Autodesk Fusion 360 part; units mm, degrees
(part 8 of 8)
equation "d2179 = ( BaseY + Depth - 12 mm )"
equation "d2180 = -( -( UpperDeckHeight - PanHeight - 8 mm ) )"
equation "d2181 = TowerFrame"
equation "d2183 = UpperDeckHeight - PanHeight"
equation "d2185 = ( BaseX ) + ( ( TowerFrame - 5 mm ) / 2 )"
equation "d2186 = ( BaseY + 8 mm ) - ( 2.5 mm )"
equation "d2189 = PegHeight"
equation "d2191 = UpperDeckHeight - PanHeight"
equation "d2193 = ( BaseX ) + ( ( TowerFrame - 5 mm ) / 2 )"
equation "d2194 = ( BaseY + Depth - 8 mm ) - ( 2.5 mm )"
equation "d2197 = PegHeight"
equation "d2201 = BaseX + TowerWidth - TowerFrame"
equation "d2202 = BaseY"
equation "d2203 = TowerFrame"
equation "d2204 = Depth"
equation "d2205 = UpperDeckHeight - PanHeight"
equation "d2207 = BaseX + TowerWidth - TowerFrame"
equation "d2209 = -( -( 8 mm ) )"
equation "d2210 = ( BaseY + 12 mm )"
equation "d2211 = ( BaseY + Depth - 12 mm )"
equation "d2212 = -( -( UpperDeckHeight - PanHeight - 8 mm ) )"
equation "d2213 = TowerFrame"
equation "d2215 = UpperDeckHeight - PanHeight"
equation "d2217 = ( BaseX + TowerWidth - TowerFrame ) + ( ( TowerFrame - 5 mm ) / 2 )"
equation "d2218 = ( BaseY + 8 mm ) - ( 2.5 mm )"
equation "d2221 = PegHeight"
equation "d2223 = UpperDeckHeight - PanHeight"
equation "d2225 = ( BaseX + TowerWidth - TowerFrame ) + ( ( TowerFrame - 5 mm ) / 2 )"
equation "d2226 = ( BaseY + Depth - 8 mm ) - ( 2.5 mm )"
equation "d2229 = PegHeight"
equation "d2231 = UpperDeckHeight - PanHeight"
equation "d2233 = ( BaseX + ( TowerFrame - 5 mm ) / 2 ) - ( FitClearance )"
equation "d2234 = ( BaseY + 8 mm ) - ( 2.5 mm + FitClearance )"
equation "d2235 = 5 mm + 2 * FitClearance"
equation "d2236 = 5 mm + 2 * FitClearance"
equation "d2237 = PegHeight + 0.3 mm"
equation "d2239 = UpperDeckHeight - PanHeight"
equation "d2241 = ( BaseX + ( TowerFrame - 5 mm ) / 2 ) - ( FitClearance )"
equation "d2242 = ( BaseY + Depth - 8 mm ) - ( 2.5 mm + FitClearance )"
equation "d2243 = 5 mm + 2 * FitClearance"
equation "d2244 = 5 mm + 2 * FitClearance"
equation "d2245 = PegHeight + 0.3 mm"
equation "d2247 = UpperDeckHeight - PanHeight"
equation "d2249 = ( BaseX + TowerWidth - TowerFrame + ( TowerFrame - 5 mm ) / 2 ) - ( FitClearance )"
equation "d2250 = ( BaseY + 8 mm ) - ( 2.5 mm + FitClearance )"
equation "d2251 = 5 mm + 2 * FitClearance"
equation "d2252 = 5 mm + 2 * FitClearance"
equation "d2253 = PegHeight + 0.3 mm"
equation "d2255 = UpperDeckHeight - PanHeight"
equation "d2257 = ( BaseX + TowerWidth - TowerFrame + ( TowerFrame - 5 mm ) / 2 ) - ( FitClearance )"
equation "d2258 = ( BaseY + Depth - 8 mm ) - ( 2.5 mm + FitClearance )"
equation "d2259 = 5 mm + 2 * FitClearance"
equation "d2260 = 5 mm + 2 * FitClearance"
equation "d2261 = PegHeight + 0.3 mm"
equation "d2265 = BaseX + LeftRun + FaucetGap + RightRun + 20 mm + 0 mm"
equation "d2266 = BaseY"
equation "d2273 = ( BaseX + LeftRun + FaucetGap + RightRun + 20 mm + 0 mm ) + ( ( 24 mm - ( PegSize + 2 * ( FitClearance - 0.05 mm ) ) ) / 2 )"
equation "d2274 = BaseY + ( 24 mm - ( PegSize + 2 * ( FitClearance - 0.05 mm ) ) ) / 2"
equation "d2275 = PegSize + 2 * ( FitClearance - 0.05 mm )"
equation "d2276 = PegSize + 2 * ( FitClearance - 0.05 mm )"
equation "d2277 = PegHeight + 0.3 mm"
equation "d2281 = BaseX + LeftRun + FaucetGap + RightRun + 20 mm + 30 mm"
equation "d2282 = BaseY"
equation "d2289 = ( BaseX + LeftRun + FaucetGap + RightRun + 20 mm + 30 mm ) + ( ( 24 mm - ( PegSize + 2 * ( FitClearance ) ) ) / 2 )"
equation "d2290 = BaseY + ( 24 mm - ( PegSize + 2 * ( FitClearance ) ) ) / 2"
equation "d2291 = PegSize + 2 * ( FitClearance )"
equation "d2292 = PegSize + 2 * ( FitClearance )"
equation "d2293 = PegHeight + 0.3 mm"
equation "d2297 = BaseX + LeftRun + FaucetGap + RightRun + 20 mm + 60 mm"
equation "d2298 = BaseY"
equation "d2305 = ( BaseX + LeftRun + FaucetGap + RightRun + 20 mm + 60 mm ) + ( ( 24 mm - ( PegSize + 2 * ( FitClearance + 0.05 mm ) ) ) / 2 )"
equation "d2306 = BaseY + ( 24 mm - ( PegSize + 2 * ( FitClearance + 0.05 mm ) ) ) / 2"
equation "d2307 = PegSize + 2 * ( FitClearance + 0.05 mm )"
equation "d2308 = PegSize + 2 * ( FitClearance + 0.05 mm )"
equation "d2309 = PegHeight + 0.3 mm"
named bodies: "L1_DrainPan", "L1_RemovableGrate", "L1_Foot_00", "L1_Foot_01", "L1_Foot_10", "L1_Foot_11", "L2_DrainPan", "L2_RemovableGrate", "L2_Foot_00", "L2_Foot_01", "L2_Foot_10", "L2_Foot_11", "R1_DrainPan", "R1_RemovableGrate", "R1_Foot_00", "R1_Foot_01", "R1_Foot_10", "R1_Foot_11", "R2_DrainPan", "R2_RemovableGrate", "R2_Foot_00", "R2_Foot_01", "R2_Foot_10", "R2_Foot_11", "LS_DrainPan", "LS_RemovableGrate", "LS_Foot_00", "LS_Foot_01", "LS_Foot_10", "LS_Foot_11", "RS_DrainPan", "RS_RemovableGrate", "RS_Foot_00", "RS_Foot_01", "RS_Foot_10", "RS_Foot_11", "UP_DrainPan", "UP_RemovableGrate", "Tower_SideFrame_1", "Tower_SideFrame_2", "FIT_Tight", "FIT_Nominal", "FIT_Loose"
